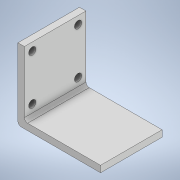
# Autodesk Inventor part: L_connector_actuators_endeffector
Saved by Autodesk Inventor 2021 (Build 250183000, 183)
## iProperties
Created: 2020-05-19
Part Number: L_connector_actuators_endeffector
Material: Generic
Document SubType Name: Modeling
Designer: Motius
Density: 1 g/cm^3
Appearance: Default
Author: Motius
Autodesk Inventor part; units mm, degrees
ref_plane "YZ Plane" through (0, 0, 0) normal (1, 0, 0) x (0, 1, 0)
ref_plane "XZ Plane" through (0, 0, 0) normal (0, 1, 0) x (-1, 0, 0)
ref_plane "XY Plane" through (0, 0, 0) normal (0, 0, 1) x (1, 0, 0)
sketch "Sketch1" plane through (0, 0, 0) normal (0, 0, 1) x (1, 0, 0)
  line L0 (-16.6971, 0) -> (55.2828, 0) construction
  line L1 (0, 46.8828) -> (0, -15.2971) construction
  line L2 (-6, 38) -> (-6, -4)
  line L3 (-4, -6) -> (45, -6)
  line L4 (45, -6) -> (45, -2)
  line L5 (45, -2) -> (0, -2)
  line L6 (-2, 0) -> (-2, 38)
  line L7 (-2, 38) -> (-6, 38)
  arc A0 (-2, 0) -> (0, -2) centre (0, 0) ccw
  arc A1 (-6, -4) -> (-4, -6) centre (-4, -4) ccw
  dimension "d0" = 2
  dimension "d1" = 4
  dimension "d2" = 4
  dimension "d3" = 38
  dimension "d5" = 45
  constraints: 12 end point, 4 point on circle, 4 tangent, 3 perpendicular, 2 centre point, 2 point on line, 1 equal radius, 1 horizontal, 1 parallel, 1 vertical
  measures "d0" radius of A0
  measures "d1" distance of L6.end L2.start
  measures "d2" distance of L3.end L4.end
  measures "d3" distance from line of L6.start L7
  measures "d5" distance from line of L4 L5.end
extrude "Extrusion1" add sketch "Sketch1" along normal mid plane 38
sketch "Sketch2" plane through (-2, 0, 19) normal (1, 0, 0) x (0, 0, -1)
  line L0 (0, 38) -> (38, 38) construction
  line L1 (0, 0) -> (0, 38) construction
  line L2 (38, 0) -> (0, 0) construction
  line L3 (38, 38) -> (38, 0) construction
  line L4 (0, 0) -> (0, 38) construction
  line L5 (0, 19) -> (38, 19) construction
  line L6 (19, 0) -> (19, 38) construction
  line L7 (0, 38) -> (38, 38) construction
  line L8 (4.858, 4.858) -> (33.142, 4.858) construction
  line L9 (33.142, 4.858) -> (33.142, 33.142) construction
  line L10 (33.142, 33.142) -> (4.858, 33.142) construction
  line L11 (4.858, 33.142) -> (4.858, 4.858) construction
  dimension "d8" = 28.284
  dimension "d9" = 28.284
  constraints: 12 end point, 4 coincident, 3 midpoint, 2 parallel, 1 horizontal, 1 perpendicular, 2 other
  measures "d8" distance of L10.end L8.start
  measures "d9" distance of L8.start L8.end
hole "Hole1" at (-2, 4.858, 14.142) at (-2, 33.142, 14.142) at (-2, 4.858, -14.142) at (-2, 33.142, -14.142) direction (-1, 0, 0) diameter 4.5 end through all clearance for "Socket Head Cap Screw" size "M4" standard "Ansi Metric M Profile"
equation "\"d9\" = d8"
body "Solid1"
